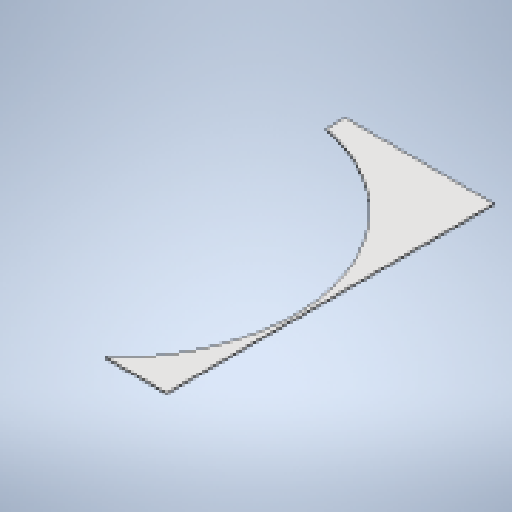
# Autodesk Inventor part: TRM 013 top main
Saved by Autodesk Inventor 2025 (Build 290162010, 162A)
## iProperties
Created: 2024-08-07
Part Number: TRM 013 top main
Material: AISI 304
Document SubType Name: Sheet Metal
Designer: pokla
Density: 8.02768 g/cm^3
Flat Pattern Width: 25 cm
Flat Pattern Length: 55 cm
Flat Pattern Area: 1375 cm^2
Sheet Metal Rule: AISI304 2mm Die16
Sheet Metal Width: 250,000 mm
Sheet Metal Length: 550,000 mm
Sheet Metal Area: 137500,000 mm^2
Appearance: Default
Stock Number: ТРМ 013 верх основное
Author: pokla
Autodesk Inventor part; units mm, degrees
ref_plane "YZ Plane" through (0, 0, 0) normal (1, 0, 0) x (0, 1, 0)
ref_plane "XZ Plane" through (0, 0, 0) normal (0, 1, 0) x (-1, 0, 0)
ref_plane "XY Plane" through (0, 0, 0) normal (0, 0, 1) x (1, 0, 0)
sketch "Sketch1" plane through (0, 0, 0) normal (0, 0, 1) x (1, 0, 0)
  line L0 (-125, -275) -> (125, -275)
  line L1 (125, -275) -> (125, 275)
  line L2 (125, 275) -> (-125, 275)
  line L3 (-125, 275) -> (-125, -275)
  line L4 (-125, -275) -> (125, 275) construction
  line L5 (125, -275) -> (-125, 275) construction
  arc A0 (-17.185, -275) -> (-125, 229.612) centre (-224.5981, -55.4919) ccw
  point P0 (0, 0)
  dimension "d22" = 550
  dimension "d23" = 250
  dimension "d24" = 302
  dimension "d25" = 45.388
  dimension "d26" = 142.185
  measures "d22" distance between parallel lines of L0 L2
  measures "d23" distance between parallel lines of L1 L3
  measures "d24" radius of A0
  measures "d25" distance of L2.end A0.end
  measures "d26" distance of L0.end A0.start
extrude "Plate1" add sketch "Sketch1" along normal blind 2 contours A0 L3 L2 L1 L0
sketch "Sketch2" plane through (0, 0, 0) normal (0, 0, -1) x (-1, 0, 0)
  line L0 (-105, 255) -> (95, 255) construction
  line L1 (95, 255) -> (95, 235) construction
  line L2 (95, 235) -> (-105, 235) construction
  line L3 (-105, 235) -> (-105, 255) construction
  line L4 (-125, 275) -> (125, 275) projected
  line L5 (-125, -275) -> (-125, 275) projected
  point P0 (0, 0)
  dimension "d6" = 200
  dimension "d9" = 20
  dimension "d10" = 20
  dimension "d11" = 20
  constraints: 2 other
  measures "d6" distance of L0.start L0.end
  measures "d9" distance of L0.end L1.end
  measures "d10" distance between parallel lines of L4 L0
  measures "d11" distance between parallel lines of L5 L3
mark "Mark1"
equation "\"d2\" = Thickness"
equation "\"BendReliefWidth\" = Thickness"
equation "\"BendReliefDepth\" = 0.5 * Thickness"
equation "\"CornerReliefSize\" = 4 * Thickness"
equation "\"MinimumRemnant\" = 2 * Thickness"
equation "\"TransitionRadius\" = BendRadius"
equation "\"JacobiRadiusSize\" = BendRadius"
equation "\"GapSize\" = Thickness"
equation "\"Thickness\" = 2"
equation "\"BendRadius\" = 2.75"
body "Solid1"
